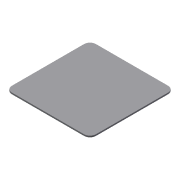
# Autodesk Inventor part: 00_Baseplate_Axiotech
Saved by Autodesk Inventor 2019 (Build 230136000, 136)
## iProperties
Created: 2019-05-20
Part Number: 00_Baseplate_Axiotech
Material: Generic
Document SubType Name: Modeling
Designer: diederichbenedict
Density: 1 g/cm^3
Appearance: Default
Author: diederichbenedict
Autodesk Inventor part; units mm, degrees
ref_plane "YZ Plane" through (0, 0, 0) normal (1, 0, 0) x (0, 1, 0)
ref_plane "XZ Plane" through (0, 0, 0) normal (0, 1, 0) x (-1, 0, 0)
ref_plane "XY Plane" through (0, 0, 0) normal (0, 0, 1) x (1, 0, 0)
sketch "Sketch1" plane through (0, 0, 0) normal (0, 1, 0) x (-1, 0, 0)
  line L0 (-49.5, -57.5) -> (49.5, -57.5)
  line L1 (57.5, -49.5) -> (57.5, 49.5)
  line L2 (49.5, 57.5) -> (-49.5, 57.5)
  line L3 (-57.5, 49.5) -> (-57.5, -49.5)
  line L4 (-57.5, -57.5) -> (57.5, 57.5) construction
  line L5 (57.5, -57.5) -> (-57.5, 57.5) construction
  arc A0 (57.5, 49.5) -> (49.5, 57.5) centre (49.5, 49.5) ccw
  arc A1 (-49.5, 57.5) -> (-57.5, 49.5) centre (-49.5, 49.5) ccw
  arc A2 (-57.5, -49.5) -> (-49.5, -57.5) centre (-49.5, -49.5) ccw
  arc A3 (49.5, -57.5) -> (57.5, -49.5) centre (49.5, -49.5) ccw
  point P0 (0, 0)
  dimension "d0" = 115
  dimension "d1" = 115
  dimension "d2" = 8
  constraints: 12 end point, 8 point on circle, 8 point on line, 8 tangent, 4 centre point, 3 equal radius, 2 midpoint, 2 parallel, 1 horizontal, 1 perpendicular
  measures "d0" distance of L5.end L4.end
  measures "d1" distance of L4.end L5.start
  measures "d2" radius of A0
extrude "Extrusion1" add sketch "Sketch1" along normal blind 2
body "Solid1"
